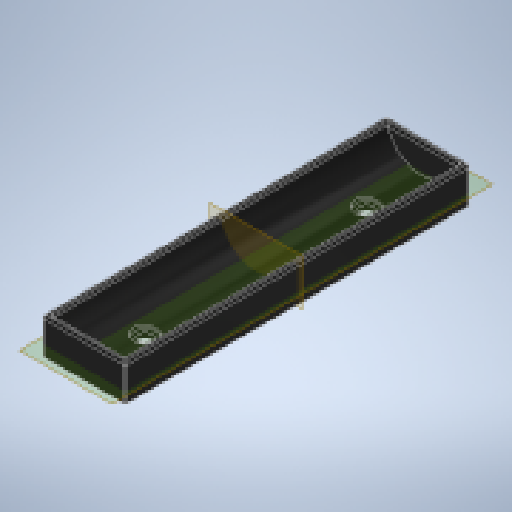
# Autodesk Inventor part: Disk_Holder
Saved by Autodesk Inventor 2025.1 (Build 291241020, 241B)
## iProperties
Created: 2024-11-14
Part Number: Disk_Holder
Material: PC/ABS Plastic
Document SubType Name: Modeling
Designer: leon-
Density: 1.1 g/cm^3
Appearance: Smooth - Black
Author: leon-
## iProperties of the stored document Disk_Holder_3DPrint.ipt
Created: 2024-11-19
Part Number: Disk_Holder_3DPrint
Material: Generic
Document SubType Name: Modeling
Designer: leon-
Density: 1 g/cm^3
Appearance: Default
Author: leon-
Autodesk Inventor part; units mm, degrees
ref_plane "YZ Plane" through (0, 0, 0) normal (1, 0, 0) x (0, 1, 0)
ref_plane "XZ Plane" through (0, 0, 0) normal (0, 1, 0) x (-1, 0, 0)
ref_plane "XY Plane" through (0, 0, 0) normal (0, 0, 1) x (1, 0, 0)
sketch "Sketch3" plane through (0, 0, 0) normal (0, 0, 1) x (1, 0, 0)
  line L0 (-19, 0) -> (19, 0)
  arc A0 (-16, 15.9689) -> (16, 15.9689) centre (0, 20) ccw
  line L1 (0, -4) -> (0, 24) projected
  line L2 (-26.6, 0) -> (26.6, 0) projected
  line L3 (-16, 15.9689) -> (-19, 15.9689)
  line L4 (-19, 15.9689) -> (-19, 0)
  line L5 (16, 15.9689) -> (19, 15.9689)
  line L6 (19, 15.9689) -> (19, 0)
  point P0 (0, 0)
  point P1 (-17.5, 15.9689)
  point P2 (17.5, 15.9689)
  dimension "d6" = 16.5
  dimension "d9" = 20
  dimension "d12" = 38
  dimension "d13" = 3
  dimension "d14" = 3
  constraints: 10 end point, 3 horizontal, 2 midpoint, 2 point on circle, 2 vertical, 1 centre point, 1 collinear, 1 horizontal alignment, 1 point on line
  measures "d6" radius of A0
  measures "d9" distance from line of L0 A0.centre
  measures "d12" distance of L0.start L0.end
  measures "d13" distance of L5.start L5.end
  measures "d14" distance of L3.start L3.end
extrude "Extrusion3" add sketch "Sketch3" along normal blind 150
ref_plane "Work Plane1" through (0, 0, 75) normal (0, 0, 1) x (1, 0, 0)
sketch "Sketch4" plane through (0, 0, 0) normal (0, 0, -1) x (-1, 0, 0)
  line L0 (-19, 0) -> (-19, 15.9689) projected
  line L1 (19, 15.9689) -> (19, 0) projected
  line L2 (-19, 15.9689) -> (19, 15.9689)
  line L3 (19, 15.9689) -> (19, 0)
  line L4 (19, 0) -> (-19, 0)
  line L5 (-19, 0) -> (-19, 15.9689)
  point P0 (0, 0)
  point P1 (19, 15.9689)
  constraints: 8 end point, 2 parallel, 1 horizontal, 1 perpendicular
extrude "Extrusion4" add sketch "Sketch4" along normal blind 3
mirror "Mirror1" about plane through (0, 0, 75) normal (0, 0, 1) of "Extrusion4"
fillet "Fillet1" radius 1 12 edges at (-16, 15.9689, 75) (-19, 15.9689, 75) (19, 15.9689, 75) (16, 15.9689, 75) (0, 15.9689, 150) (0, 15.9689, 153) (0, 15.9689, -3) (0, 15.9689, 0) (19, 7.9844, -3) (19, 7.9844, 153) (-19, 7.9844, 153) (-19, 7.9844, -3)
ref_plane "Work Plane2" through (-18, 5, -3) normal (0, -1, 0) x (1, 0, 0)
sketch "Sketch5" plane through (-18, 5, -3) normal (0, -1, 0) x (1, 0, 0)
  line L0 (-1, 1) -> (-1, 155) projected
  line L1 (0, 156) -> (36, 156) projected
  line L2 (36, 0) -> (0, 0) projected
  point P0 (18, 3)
  point P1 (18, 128)
  point P2 (18, 28)
  dimension "d20" = 19
  dimension "d21" = 100
  dimension "d22" = 28
  dimension "d23" = 28
  constraints: 1 vertical alignment
  measures "d20" distance from line of L0 point (18, 128)
  measures "d21" distance of point (18, 28) point (18, 128)
  measures "d22" distance from line of L1 point (18, 128)
  measures "d23" distance from line of L2 point (18, 28)
hole "Hole1" at (0, 5, 125) at (0, 5, 25) direction (0, -1, 0) diameter 6 end through all counterbore diameter 10 counterbore depth 2.5
body "Solid2"
